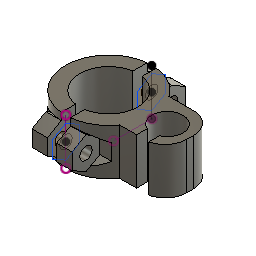
wire clip v2 (Autodesk Fusion 360 design; units mm, degrees)
Autodesk Fusion 360 part; units mm, degrees
note: some values were not read from the file. Chosen so that the rebuilt part matches the saved one: which bodies a step acts on; which face or edge a step refers to. Set by a fixed rule: which sketch regions a step uses.
sketch "Sketch1" plane through (0, 0, 0) normal (0, 1, 0) x (1, 0, 0)
  circle A0 centre (0, 0) radius 9.4
  circle A1 centre (0, 0) radius 14
  line L0 (-18.033, 1.5) -> (-9.2795, 1.5)
  line L1 (-19.033, -1.5) -> (-9.2795, -1.5)
  line L2 (0, 0) -> (-36.033, 0) construction
  line L3 (11.4891, -8) -> (26.4306, -8)
  line L4 (26.4306, -8) -> (26.4306, 8)
  line L5 (26.4306, 8) -> (11.4891, 8)
  circle A2 centre (19, 0) radius 5
  line L6 (-1.5, 22) -> (-1.5, -24.4186)
  line L7 (1.5, 22) -> (1.5, -24)
  line L8 (0, 0) -> (0, 21) construction
  line L9 (21, -4.5826) -> (21, -8)
  line L10 (17, -4.5826) -> (17, -8)
  dimension "d1" = 18.8
  dimension "d2" = 28
  dimension "d5" = 1.5
  dimension "d6" = 1.5
  dimension "d23" = 8
  dimension "d24" = 8
  dimension "d64" = 10
  dimension "d65" = 19
  dimension "d72" = 1.5
  dimension "d73" = 1.5
  dimension "d89" = 2
  dimension "d90" = 2
  measures "d1" diameter of A0
  measures "d2" diameter of A1
  measures "d5" distance of A0.centre L0
  measures "d6" distance of A0.centre L1
  measures "d23" distance of A0.centre L3
  measures "d24" distance of A0.centre L5
  measures "d64" diameter of A2
  measures "d65" distance of A0.centre
  measures "d72" distance of A0.centre L6
  measures "d73" distance of A0.centre L7
  measures "d89" distance of L9
  measures "d90" distance of L10
extrude "Extrude1" add sketch "Sketch1" along normal blind 18 contours A0 A1 L0 L6 | A0 A1 L1 L6 | A0 A1 L6 L7 | A0 A1 L6 L7 | A0 A1 L7 | A1 L3 L4 L5 A2 L9 | A1 L3 A2 L10 makes body 1
sketch "Sketch2" plane through (0, 0, 0) normal (0, 0, 1) x (1, 0, 0)
  circle A0 centre (-13.9194, 9) radius 2
  line L0 (-8.9483, 11.8701) -> (-13.9194, 14.7402)
  line L1 (-13.9194, 14.7402) -> (-18.8906, 11.8701)
  line L2 (-18.8906, 11.8701) -> (-18.8906, 6.1299)
  line L3 (-18.8906, 6.1299) -> (-13.9194, 3.2598)
  line L4 (-13.9194, 3.2598) -> (-8.9483, 6.1299)
  line L5 (-8.9483, 6.1299) -> (-8.9483, 11.8701)
  line L6 (-13.9194, 0) -> (-13.9194, 18)
  dimension "d7" = 4
  measures "d7" diameter of A0
sketch "Sketch4" plane through (0, 0, 0) normal (0, 1, 0) x (1, 0, 0)
  line L0 (22.5, 2.5981) -> (18, 5.1962)
  line L1 (18, 5.1962) -> (13.5, 2.5981)
  line L2 (13.5, 2.5981) -> (13.5, -2.5981)
  line L3 (13.5, -2.5981) -> (18, -5.1962)
  line L4 (18, -5.1962) -> (22.5, -2.5981)
  line L5 (22.5, -2.5981) -> (22.5, 2.5981)
  line L6 (13.5, 10.5) -> (13.5, -10.5)
  line L7 (13.5, -10.5) -> (15.2929, -10.5)
  line L8 (15.2929, -10.5) -> (18.7929, -7)
  line L9 (18.7929, -7) -> (29.5, -7)
  line L10 (29.5, -7) -> (29.5, 7)
  line L11 (29.5, 7) -> (18.7929, 7)
  line L12 (18.7929, 7) -> (15.2929, 10.5)
  line L13 (15.2929, 10.5) -> (13.5, 10.5)
  line L14 (18, 5.1962) -> (13.5, 5.1962)
  line L15 (18, -5.1962) -> (13.5, -5.1962)
  circle A0 centre (18, 0) radius 2
  circle A1 centre (18, 0) radius 3.25
  dimension "d69" = 4
  dimension "d70" = 6.5
  measures "d69" diameter of A0
  measures "d70" diameter of A1
extrude "Extrude2" cut sketch "Sketch2" along normal mid plane 38 contours A0 L6 | A0 L6 bodies 1
extrude "Extrude3" cut sketch "Sketch2" along normal mid plane 40 contours A0 L1 L2 L3 L6
extrude "Extrude4" add sketch "Sketch2" along normal mid plane 13 contours A0 L0 L4 L5 L6 | A0 L1 L2 L3 L6 makes body 2
extrude "Extrude5" cut sketch "Sketch2" along normal mid plane 3 contours A0 L0 L4 L5 L6 | A0 L1 L2 L3 L6 bodies 2 makes body 3 at (-17.9002, 9, 1.5)
extrude "Extrude6" cut sketch "Sketch1" along normal blind 25 contours A0 L6 | A0 L6 L7 | A0 L7 bodies 1 2 3
extrude "Extrude7" add sketch "Sketch1" along normal blind 3 contours A0 L6 | A0 A1 L0 L6 | A0 A1 L0 L1 | A0 A1 L1 L6 | A0 A1 L6 L7 | A0 L6 L7 | A0 A1 L6 L7 | A0 A1 L7 | A0 L7 | A1 L3 L4 L5 A2 L9 | A1 L3 A2 L10 | L3 A2 L9 L10 bodies 3 makes body 4
extrude "Extrude8" add sketch "Sketch4" along normal mid plane 16 separate body contours L0 L1 L2 L3 L4 L5 L6 | L0 L4 L5 L6 L7 L8 L9 L10 L11 L12 L13 L14 L15 | L1 L6 L14 | L3 L6 L15 | A1 makes body 5
extrude "Extrude9" cut sketch "Sketch4" along normal mid plane 3.4 contours L0 L1 L2 L3 L4 L5 L6 | L1 L6 L14 | L3 L6 L15 | A1 bodies 5
extrude "Extrude10" cut sketch "Sketch4" against normal blind 11 contours A1 bodies 5
sketch "Sketch3" plane through (29.5, 0, 0) normal (1, 0, 0) x (0, 0, -1)
  line L0 (7, -8) -> (7, 8)
  line L1 (7, 8) -> (-7, 8)
  line L2 (-7, 8) -> (-7, -8)
  line L3 (-7, -8) -> (7, -8)
  line L4 (-5.75, 1) -> (5.75, 1)
  line L5 (5.75, 1) -> (5.75, 3)
  line L6 (5.75, 3) -> (3.5, 3)
  line L7 (3.5, 3) -> (3.5, 6)
  line L8 (3.5, 6) -> (-3.5, 6)
  line L9 (-3.5, 6) -> (-3.5, 3)
  line L10 (-3.5, 3) -> (-5.75, 3)
  line L11 (-5.75, 3) -> (-5.75, 1)
  line L12 (7, -8) -> (7, 8)
  line L13 (7, 8) -> (-7, 8)
  line L14 (-7, 8) -> (-7, -8)
  line L15 (-7, -8) -> (7, -8)
  dimension "d45" = 5.75
  dimension "d46" = 5.75
  dimension "d47" = 3.5
  dimension "d48" = 3.5
  dimension "d49" = 5
  dimension "d50" = 2
  dimension "d51" = 2
  dimension "d71" = 9
  measures "d45" distance of L11 origin
  measures "d46" distance of L5 origin
  measures "d47" distance of L9 origin
  measures "d48" distance of L7 origin
  measures "d49" distance of L4 L8
  measures "d71" distance of L3 L4
extrude "Extrude11" cut sketch "Sketch3" against normal blind 6 contours L4 L5 L6 L7 L8 L9 L10 L11 bodies 5
extrude "Extrude12" add sketch "Sketch1" along normal blind 15 separate body contours A0 A1 L0 L6 | A0 A1 L0 L1 | A0 A1 L1 L6 | A0 A1 L7 | A1 L3 L4 L5 A2 L9 | A1 L3 A2 L10 makes body 6 at (16.7476, 5, -4.4639) makes body 7 at (-10.8601, 10, -8.8351)
ref_plane "WorkPlane1" through (0, 0, -10.5) normal (1, 0, 0) x (0, 0, -1)
sketch "Sketch5" plane through (0, 0, -10.5) normal (1, 0, 0) x (0, 0, -1)
  circle A0 centre (3.4194, 7.5) radius 2
  line L0 (3.4194, 0) -> (3.4194, 15)
  line L1 (-1.0777, 4.9036) -> (3.4194, 2.3072)
  line L2 (3.4194, 2.3072) -> (7.9165, 4.9036)
  line L3 (7.9165, 4.9036) -> (7.9165, 10.0964)
  line L4 (7.9165, 10.0964) -> (3.4194, 12.6928)
  line L5 (3.4194, 12.6928) -> (-1.0777, 10.0964)
  line L6 (-1.0777, 10.0964) -> (-1.0777, 4.9036)
  circle A1 centre (-24.4194, 7.5) radius 2
  line L7 (-24.4194, 0) -> (-24.4194, 15)
  line L8 (-19.9194, 10.0981) -> (-24.4194, 12.6962)
  line L9 (-24.4194, 12.6962) -> (-28.9194, 10.0981)
  line L10 (-28.9194, 10.0981) -> (-28.9194, 4.9019)
  line L11 (-28.9194, 4.9019) -> (-24.4194, 2.3038)
  line L12 (-24.4194, 2.3038) -> (-19.9194, 4.9019)
  line L13 (-19.9194, 4.9019) -> (-19.9194, 10.0981)
  line L14 (3.5, 0) -> (-9, 0)
  dimension "d77" = 4
  dimension "d78" = 4
  measures "d77" diameter of A0
  measures "d78" diameter of A1
extrude "Extrude13" cut sketch "Sketch5" along normal mid plane 24 bodies 6 7
extrude "Extrude17" cut sketch "Sketch5" along normal blind 15 contours A0 L0 | A0 L0 | A1 L7 | A1 L7 bodies 6
extrude "Extrude14" add sketch "Sketch5" along normal mid plane 13 contours A0 L0 L2 L3 L4 | A0 L0 L1 L5 L6 | A1 L7 L8 L12 L13 | A1 L7 L9 L10 L11 bodies 6 7
extrude "Extrude15" cut sketch "Sketch5" along normal mid plane 3 contours A0 L0 L2 L3 L4 | A0 L0 L1 L5 L6 | A1 L7 L8 L12 L13 | A1 L7 L9 L10 L11 bodies 6 makes body 8 at (16.7476, 5, -4.4639)
fillet "Fillet2" radius 7 2 edges at (26.4306, 7.5, -8) (26.4306, 7.5, 8) on bodies 8
copy_body "Body->Comp3" bodies 6 removing the originals makes body 9 in component "wire holder base"
copy_body "Body->Comp4" bodies 8 removing the originals makes body 10 in component "wire holder"
extrude "Extrude16" [suppressed]
combine "Combine1" [suppressed] in component "sencor mount horiz"
copy_body "CopyPasteBodies1" [suppressed]
copy_body "Body->Comp1" [suppressed] in component "sensor mount"
copy_body "Body->Comp2" [suppressed] in component "Sensor Holder"
component "wire holder base" placed x (1, 0, 0) y (0, 1, 0) z (0, 0, 1) at (0, 0, 0)
component "wire holder" placed x (1, 0, 0) y (0, 1, 0) z (0, 0, 1) at (0, 0, 0)
hidden bodies 1 2 3 4 5
named bodies: "Sensor Holder", "sensor mount"
